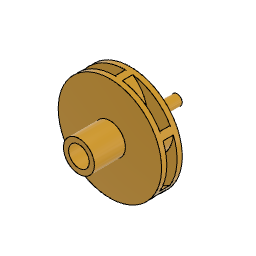
_IMPELLER.7104f649-9f54-4860-be15-78095c53e5d1 (Autodesk Fusion 360 design; units mm, degrees)
Autodesk Fusion 360 part; units mm, degrees
sketch "I Base" plane through (0, 0, 0) normal (0, 1, 0) x (1, 0, 0)
  circle A0 centre (0, 0) radius 50
  circle A1 centre (0, 0) radius 5
  circle A2 centre (0, 0) radius 2.5
  dimension "d1" = 100
  dimension "d47" = 10
  dimension "d48" = 5
  constraint coincident A0.centre A1.centre
  constraint concentric A0 A1
  constraint concentric A0 A2
  measures "d1" diameter of A0
  measures "d47" diameter of A1
  measures "d48" diameter of A2
extrude "Extrude1" add sketch "I Base" along normal blind 5 contours A0 | A1 | A2 makes body 1
sketch "Blade" plane through (0, 0, 0) normal (0, -1, 0) x (1, 0, 0)
  circle A0 centre (0, 0) radius 50
  arc A1 (8.9565, 0.6501) -> (0, 50) centre (-11.7219, 22.3849) ccw
  arc A2 (11.0244, -1.5234) -> (7.0955, 49.494) centre (-11.7219, 22.3849) ccw
  arc A3 (8.9565, 0.6501) -> (11.0244, -1.5234) centre (9.9905, -0.4367) ccw
  line L0 (0, 50) -> (-12.3857, 55.2574) construction
  line L1 (-12.3857, 55.2574) -> (0, 50) construction
  line L2 (-12.7386, 50) -> (0, 50) construction
  circle A4 centre (0, 0) radius 10 construction
  circle A5 centre (0, 0) radius 10 construction
  arc A6 (3.9153, 8.0816) -> (-43.3013, 25) centre (-25.2468, 1.0409) ccw
  arc A7 (6.8315, 8.7857) -> (-39.3153, 30.8919) centre (-25.2468, 1.0409) ccw
  arc A8 (3.9153, 8.0816) -> (6.8315, 8.7857) centre (5.3734, 8.4337) ccw
  circle A9 centre (0, 0) radius 10 construction
  arc A10 (-5.0412, 7.4316) -> (-43.3013, -25) centre (-13.5249, -21.3439) ccw
  arc A11 (-4.1929, 10.3091) -> (-46.4108, -18.6021) centre (-13.5249, -21.3439) ccw
  arc A12 (-5.0412, 7.4316) -> (-4.1929, 10.3091) centre (-4.6171, 8.8703) ccw
  circle A13 centre (0, 0) radius 10 construction
  arc A14 (-8.9565, -0.6501) -> (0, -50) centre (11.7219, -22.3849) ccw
  arc A15 (-11.0244, 1.5234) -> (-7.0955, -49.494) centre (11.7219, -22.3849) ccw
  arc A16 (-8.9565, -0.6501) -> (-11.0244, 1.5234) centre (-9.9905, 0.4367) ccw
  circle A17 centre (0, 0) radius 10 construction
  arc A18 (-3.9153, -8.0816) -> (43.3013, -25) centre (25.2468, -1.0409) ccw
  arc A19 (-6.8315, -8.7857) -> (39.3153, -30.8919) centre (25.2468, -1.0409) ccw
  arc A20 (-3.9153, -8.0816) -> (-6.8315, -8.7857) centre (-5.3734, -8.4337) ccw
  circle A21 centre (0, 0) radius 10 construction
  arc A22 (5.0412, -7.4316) -> (43.3013, 25) centre (13.5249, 21.3439) ccw
  arc A23 (4.1929, -10.3091) -> (46.4108, 18.6021) centre (13.5249, 21.3439) ccw
  arc A24 (5.0412, -7.4316) -> (4.1929, -10.3091) centre (4.6171, -8.8703) ccw
  dimension "d5" = 30
  dimension "d6" = 33
  dimension "d7" = 1.5
  dimension "d11" = 23
  dimension "d14" = 360
  dimension "d30" = 20
  constraint coincident A0 A1.end
  constraint concentric A1 A2
  constraint coincident A0 A2.end
  constraint vertical A1.end A0.centre
  constraint parallel L0 L1
  constraint tangent A0 L2
  constraint tangent A1 L1
  constraint coincident A0.centre A4.centre
  constraint coincident A3.centre A4
  constraint tangent A2 A3
  measures "d5" radius of A1
  measures "d6" radius of A2
  measures "d7" radius of A3
  measures "d11" angle of L1 L2
  measures "d30" diameter of A9
extrude "Extrude2" add sketch "Blade" along normal blind 10 contours A0 A22 A23 A24 | A0 A18 A19 A20 | A0 A1 A2 A3 | A0 A14 A15 A16 | A0 A6 A7 A8 | A0 A10 A11 A12 bodies 1
ref_plane "WorkPlane1" through (0, -10, 0) normal (0, 1, 0) x (0, 0, 1)
sketch "I Face" plane through (0, -10, 0) normal (0, 1, 0) x (1, 0, 0)
  circle A0 centre (0, 0) radius 50
  dimension "d18" = 100
  constraint coincident A0.centre origin
  measures "d18" diameter of A0
extrude "Extrude3" add sketch "I Face" against normal blind 5 separate body makes body 2
sketch "sharp blade" plane through (0, 0, 0) normal (1, 0, 0) x (0, 1, 0)
  line L0 (0, 0) -> (-20, 0)
  line L1 (0, 10) -> (0, 0)
  line L2 (0, 0) -> (-10, 0)
  line L3 (0, 10) -> (0, 0)
  line L4 (-10, 30) -> (-10, 0)
  arc A0 (-10, 30) -> (0, 10) centre (15, 30) ccw
  dimension "d24" = 20
  dimension "d25" = 10
  dimension "d33" = 10
  dimension "d36" = 30
  constraint coincident L0.start L1.end
  constraint horizontal L0
  constraint perpendicular L0 L1
  constraint horizontal L2
  constraint vertical L3
  constraint perpendicular L2 L4
  constraint coincident L1.start L3.start
  constraint tangent L4 A0
  measures "d24" distance of L0.start L0.end
  measures "d25" distance of L0.start L1.start
  measures "d33" distance of L0.start L4
  measures "d36" distance of L2.end L4.start
revolve "Revolve1" cut sketch "sharp blade" angle 360 about axis through (0, 0, 0) along (0, -1, 0) bodies 1
hole "Hole1" at (0, -15, 0) direction (0, 1, 0) diameter 20 depth 5 tip angle 180 bodies 2
delete_face "DeleteFace1" 1 faces at (0.4985, -13.3333, -9.9876) on bodies 2
sketch "Hole on IFace" plane through (0, -15, 0) normal (0, -1, 0) x (1, 0, 0)
  circle A0 centre (0, 0) radius 50
  circle A1 centre (0, 0) radius 10
  circle A2 centre (0, 0) radius 15
  dimension "d40" = 20
  dimension "d44" = 30
  constraint concentric A0 A1
  constraint concentric A1 A2
  measures "d40" diameter of A1
  measures "d44" diameter of A2
hole "Hole2" at (0, -15, 0) direction (0, 1, 0) diameter 20 depth 5 tip angle 180 bodies 2
combine "Combine1" operation add target body 1 tool bodies 2
extrude "Extrude4" add sketch "Hole on IFace" along normal blind 30 contours A2 bodies 1
extrude "Extrude5" add sketch "I Base" along normal blind 50 contours A1 bodies 1
extrude "Extrude8" cut sketch "I Base" along normal blind 5 contours A2 bodies 1
named bodies: "IMPELLER"
